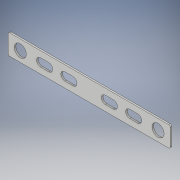
# Autodesk Inventor part: Side Plate
Saved by Autodesk Inventor 2019 (Build 230136000, 136)
## iProperties
Created: 2019-10-06
Part Number: Side Plate
Material: Generic
Document SubType Name: Modeling
Designer: robgr
Density: 1 g/cm^3
Appearance: Default
Author: robgr
Autodesk Inventor part; units mm, degrees
ref_plane "YZ Plane" through (0, 0, 0) normal (1, 0, 0) x (0, 1, 0)
ref_plane "XZ Plane" through (0, 0, 0) normal (0, 1, 0) x (-1, 0, 0)
sketch "Sketch1" plane through (0, 0, 0) normal (0, 0, 1) x (1, 0, 0)
  line L0 (-25.0719, 9.0848) -> (170.9281, 9.0848)
  line L1 (172.9281, 7.0848) -> (172.9281, -13.9152)
  line L2 (170.9281, -15.9152) -> (-25.0719, -15.9152)
  line L3 (-27.0719, -13.9152) -> (-27.0719, 7.0848)
  arc A0 (-25.0719, 9.0848) -> (-27.0719, 7.0848) centre (-25.0719, 7.0848) ccw
  arc A1 (-27.0719, -13.9152) -> (-25.0719, -15.9152) centre (-25.0719, -13.9152) ccw
  arc A2 (170.9281, -15.9152) -> (172.9281, -13.9152) centre (170.9281, -13.9152) ccw
  arc A3 (172.9281, 7.0848) -> (170.9281, 9.0848) centre (170.9281, 7.0848) ccw
  point P0 (0, 0)
  point P1 (172.9281, -15.9152)
  point P2 (172.9281, 9.0848)
  point P3 (-27.0719, -15.9152)
  dimension "d0" = 200
  dimension "d1" = 25
  dimension "d2" = 2
  constraints: 8 end point, 8 point on circle, 8 tangent, 6 point on line, 4 centre point, 3 equal radius, 2 parallel, 1 horizontal, 1 perpendicular
  measures "d0" distance of point (172.928, -15.915) point (-27.072, -15.915)
  measures "d1" distance of point (172.928, 9.085) point (172.928, -15.915)
  measures "d2" radius of A0
extrude "Extrusion1" add sketch "Sketch1" along normal blind 2
sketch "Sketch2" plane through (0, 0, 2) normal (0, 0, 1) x (1, 0, 0)
  line L0 (170.9281, -15.9152) -> (-25.0719, -15.9152) projected
  line L1 (72.9281, -15.9152) -> (72.9281, 9.0848)
  line L2 (170.9281, 9.0848) -> (-25.0719, 9.0848) projected
  line L3 (-27.0719, 7.0848) -> (-27.0719, -13.9152) projected
  line L4 (-27.0719, -3.4152) -> (172.9281, -3.4152)
  line L5 (172.9281, 7.0848) -> (172.9281, -13.9152) projected
  circle A0 centre (-12.0719, -3.4152) radius 7.5
  line L6 (7.9281, -3.4152) -> (27.9281, -3.4152) construction
  line L7 (12.9281, -8.4152) -> (22.9281, -8.4152)
  line L8 (22.9281, 1.5848) -> (12.9281, 1.5848)
  arc A1 (12.9281, 1.5848) -> (12.9281, -8.4152) centre (12.9281, -3.4152) ccw
  arc A2 (22.9281, -8.4152) -> (22.9281, 1.5848) centre (22.9281, -3.4152) ccw
  line L9 (37.9281, -3.4152) -> (57.9281, -3.4152) construction
  line L10 (42.9281, 1.5848) -> (52.9281, 1.5848)
  line L11 (52.9281, -8.4152) -> (42.9281, -8.4152)
  arc A3 (42.9281, 1.5848) -> (42.9281, -8.4152) centre (42.9281, -3.4152) ccw
  arc A4 (52.9281, -8.4152) -> (52.9281, 1.5848) centre (52.9281, -3.4152) ccw
  point P0 (0, 0)
  point P1 (17.9281, -3.4152)
  point P2 (47.9281, -3.4152)
  dimension "d5" = 15
  dimension "d6" = 15
  dimension "d7" = 20
  dimension "d8" = 10
  dimension "d9" = 20
  dimension "d10" = 30
  dimension "d11" = 25
  constraints: 20 end point, 12 point on circle, 9 point on line, 8 tangent, 6 midpoint, 5 centre point, 2 parallel
  measures "d5" diameter of A0
  measures "d6" distance from line of L3 A0.centre
  measures "d7" distance of L6.start L6.end
  measures "d8" diameter of A2
  measures "d9" distance of L9.start L9.end
  measures "d10" distance of point (17.928, -3.415) point (47.928, -3.415)
  measures "d11" distance from line of L1 point (47.928, -3.415)
extrude "Extrusion2" cut sketch "Sketch2" against normal blind 2
ref_plane "Work Plane1" through (72.9281, -13.9152, 0) normal (1, 0, 0) x (0, 0, -1)
mirror "Mirror1" about plane through (72.9281, -13.9152, 0) normal (1, 0, 0) of "Extrusion2"
body "Solid1"
